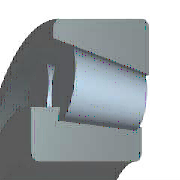
# Autodesk Inventor part: Подшипник 7205A ГОСТ 27365-87
Saved by Autodesk Inventor 2021 (Build 250183000, 183)
## iProperties
Created: 2020-01-21
Part Number: Подшипник 7205A ГОСТ 27365-87
Material: Сталь, мягкая
Description: Подшипники роликовые конические однорядные повышенной грузоподъемности
Document SubType Name: Modeling
Standard: ГОСТ 27365-87
Designer: gdevc
Standards Organization: GOST
Language: ru-RU
Size Designation: 7205A
Categories: <MemberInstance><Categories><Category DisplayName="Детали вала" InternalName="7f7aeb1f-a693-4053-b835-cee3144e0d98" Mnemonic="SHFT"><Category DisplayName="Подшипники" InternalName="242d30a3-7172-44e6-a363-b0a3d8f1b556" Mnemonic="BRNG"><CategoryParameter DisplayName="Ширина" InternalName="25fc5f6e-338b-4801-b5ed-8959743e396e" Mnemonic="wdth"/><CategoryParameter DisplayName="Обозначение размера" InternalName="2c4e891a-c8f4-49ed-a5c1-5131476c6feb" Mnemonic="sizedes"/><CategoryParameter DisplayName="Номинальная динамическая нагрузка" InternalName="440972dd-7009-4861-bd45-69ffbb461423" Mnemonic="bdynlrat"/><CategoryParameter DisplayName="Диаметр вала" InternalName="91302473-2833-4451-a660-c5d4a8d6a031" Mnemonic="shaftdia"/><CategoryParameter DisplayName="Угол касания" InternalName="aa21a452-7974-4a55-b5cf-1c2972de2aea" Mnemonic="TouchAngle"/><CategoryParameter DisplayName="Наружный диаметр" InternalName="d441686c-04bd-4681-b674-94fbc173ec23" Mnemonic="outdia"/><Category DisplayName="Подшипники роликовые" InternalName="a40a3fd7-d489-4921-9892-cb944902a182" Mnemonic="ROLLBEAR"><CategoryParameter DisplayName="Номинальная статическая нагрузка" InternalName="124ef669-bc53-497e-8b3b-9e9432584ac1" Mnemonic="bstatlrat"/><CategoryParameter DisplayName="Коэффициент радиальной динамической нагрузки при Fa/Fr &gt; e" InternalName="1feec4eb-3d91-4913-989d-fa96ab069f3d" Mnemonic="raddynfc2"/><CategoryParameter DisplayName="Коэффициент осевой динамической нагрузки при Fa/Fr &gt; e" InternalName="200b4357-faba-40fb-9da6-9412c8ddeb78" Mnemonic="axdynfc2"/><CategoryParameter DisplayName="Радиус" InternalName="2322b21e-a448-4b16-bf77-0b09a9a1e5fa" Mnemonic="rad"/><CategoryParameter DisplayName="Мин. диаметр вала" InternalName="27c639de-1f82-42cb-a17a-a84ebe509f1b" Mnemonic="minshaftdia"/><CategoryParameter DisplayName="Ограничивающая скорость смазка" InternalName="34ed7782-22cd-44b7-90f2-16a4b10c8234" Mnemonic="lubgrsp"/><CategoryParameter DisplayName="Масса" InternalName="35563771-cdde-4f36-b8ea-a6490dc90073" Mnemonic="mass"/><CategoryParameter DisplayName="Ограничивающее скорость масло" InternalName="576744bc-a99a-4f12-bf8b-8b83672ef882" Mnemonic="oilspd"/><CategoryParameter DisplayName="Коэффициент радиальной статической нагрузки" InternalName="646321f5-f93b-4aec-b962-0341aa1dcfaf" Mnemonic="raddynfc0"/><CategoryParameter DisplayName="Макс. радиус отсека скругления" InternalName="890763e8-95b6-457a-9b07-8de657924e40" Mnemonic="maxstprad"/><CategoryParameter DisplayName="Коэффициент осевой динамической нагрузки при Fa/Fr &lt;= e" InternalName="b1d498d2-5149-4618-b12c-23a3d5a7c887" Mnemonic="axdynfc1"/><CategoryParameter DisplayName="Коэффициент радиальной динамической нагрузки при Fa/Fr  &lt;= e" InternalName="b75e8b40-fb1d-483d-887b-ce2ffe1b5422" Mnemonic="raddynfc1"/><CategoryParameter DisplayName="Коэффициент трения" InternalName="ceddb76f-d381-429d-bef5-367584929fdf" Mnemonic="fricfct"/><CategoryParameter DisplayName="Коэффициент осевой статической нагрузки" InternalName="ea413b62-e115-405b-882c-23d570c3be21" Mnemonic="axdynfc0"/><CategoryParameter DisplayName="Граничное значение для определения коэффициента" InternalName="f0539972-a230-481a-8ae0-28002199c8fb" Mnemonic="limvalfac"/><CategoryParameter DisplayName="Ресурс" InternalName="f80a4cc4-8fb3-4eaa-808e-6f490e608712" Mnemonic="lifeexp"/><CategoryParameter DisplayName="Макс. диаметр отсека втулки" InternalName="feeea31f-2614-4692-af6e-a054e6e558b2" Mnemonic="maxhubdia"/><Category DisplayName="Подшипники роликовые конические" InternalName="326936b4-87e6-427a-a604-f9fe807308df" Mnemonic="RBTRB"/></Category></Category></Category><Category DisplayName="ТипДанных" InternalName="23b78d0f-2648-40c6-8793-ca6db495c9e8" Mnemonic="DATATYPE"><CategoryParameter DisplayName="ОтображаемоеИмя" InternalName="05415f3d-3907-474b-a020-eb9d644f4cf3" Mnemonic="DISPLAYNAME"/><CategoryParameter DisplayName="Стандарт" InternalName="0c0a119c-1e12-4c84-803f-101930972f5e" Mnemonic="STANDARD"/><CategoryParameter DisplayName="Наименование" InternalName="13903e3d-64b1-4950-80da-f627842ea37f" Mnemonic="DESCRIPTION"/><CategoryParameter DisplayName="Обозначение" InternalName="2675968c-4ce5-49e0-a4f5-552d29089031" Mnemonic="DESIGNATION"/><CategoryParameter DisplayName="Строка по умолчанию" InternalName="2af9ec52-faaa-4026-b378-f9fa4afca842" Mnemonic="DEFAULTROW"/><CategoryParameter DisplayName="Имя папки" InternalName="3f06958e-8713-4116-9be7-ed6184ecc97b" Mnemonic="FOLDERNAME"/><CategoryParameter DisplayName="Указатель редакций" InternalName="45a75005-10b1-4dfc-8d6d-dfe629f0b93c" Mnemonic="REVISIONGUID"/><CategoryParameter DisplayName="ИмяФайла" InternalName="8b46a4cc-9585-4fed-90c3-899f57e09a73" Mnemonic="FILENAME"/><CategoryParameter DisplayName="ОргСтанд" InternalName="8f5914e1-4693-403f-8ab5-d37768198c9d" Mnemonic="STDSORG"/><CategoryParameter DisplayName="Версия семейства" InternalName="914462f6-6e19-4b14-ba84-155b9680b1d0" Mnemonic="FAMILYREVISION"/><CategoryParameter DisplayName="Редакция стандарта" InternalName="91d5a463-65c2-4fde-b823-3b7fea5e8e17" Mnemonic="STANDARDREVISION"/><CategoryParameter DisplayName="редакция элемента" InternalName="a65d44b9-392f-4f4f-857b-e4b3d54996fe" Mnemonic="MEMBERREVISION"/><CategoryParameter DisplayName="ФорматКлипа" InternalName="bc51e27b-3422-4e78-93ef-cec197ddf230" Mnemonic="CLIPFORMAT"/><CategoryParameter DisplayName="Изготовитель" InternalName="cd6c7a72-a28a-4e50-99a9-2c7f4e13e5ad" Mnemonic="MANUFACTURER"/><CategoryParameter DisplayName="ВнутреннееИмя" InternalName="cf1d0246-76d9-4b4a-8305-fa0409afb5c1" Mnemonic="INTERNALNAME"/><CategoryParameter DisplayName="Метрическая" InternalName="e2385c5b-1ea4-4823-96a8-8de651266ec3" Mnemonic="ISMETRIC"/><Category DisplayName="Деталь" InternalName="c0e0b642-3bcb-4cc8-9e80-f96d35c4afa4" Mnemonic="PART"><CategoryParameter DisplayName="Номер детали" InternalName="016b6077-bfbe-49bd-92c9-d8d59c39c941" Mnemonic="PARTNUMBER"/><CategoryParameter DisplayName="Инвентарный номер" InternalName="4dba7c1c-e26c-444e-836c-b08b433409a8" Mnemonic="STOCKNUMBER"/><CategoryParameter DisplayName="Ключ материала" InternalName="5c9a8adb-dd2b-4535-b97f-0a94a95fe41f" Mnemonic="MATERIALKEY"/><CategoryParameter DisplayName="Материал" InternalName="818a152a-d3c3-49ca-80ee-df7d91421b8e" Mnemonic="MATERIAL"/></Category></Category></Categories><FamilyTemplate Id="Bearing GOST 27365-87"><FamilyTemplateParameters><FamilyTemplateParameter ObjectType="kUserParameterObject" ValueType="xs:double" Id="1" ObjectReferenceKey="Angle"/><FamilyTemplateParameter ObjectType="kUserParameterObject" ValueType="xs:double" Id="2" ObjectReferenceKey="B"/><FamilyTemplateParameter ObjectType="kUserParameterObject" ValueType="xs:double" Id="3" ObjectReferenceKey="C0_"/><FamilyTemplateParameter ObjectType="kUserParameterObject" ValueType="xs:double" Id="4" ObjectReferenceKey="C_"/><FamilyTemplateParameter ObjectType="kUserParameterObject" ValueType="xs:double" Id="5" ObjectReferenceKey="C__"/><FamilyTemplateParameter ObjectType="kUserParameterObject" ValueType="xs:double" Id="6" ObjectReferenceKey="d"/><FamilyTemplateParameter ObjectType="kUserParameterObject" ValueType="xs:double" Id="7" ObjectReferenceKey="D_"/><FamilyTemplateParameter ObjectType="kUserParameterObject" ValueType="xs:double" Id="8" ObjectReferenceKey="E_"/><FamilyTemplateParameter ObjectType="kUserParameterObject" ValueType="xs:double" Id="10" ObjectReferenceKey="r1_smin"/><FamilyTemplateParameter ObjectType="kUserParameterObject" ValueType="xs:double" Id="11" ObjectReferenceKey="r2_smin"/><FamilyTemplateParameter ObjectType="kUserParameterObject" ValueType="xs:double" Id="13" ObjectReferenceKey="T_"/><FamilyTemplateParameter ObjectType="kPropertyObject" ValueType="xs:string" Id="100" ObjectReferenceKey="{32853F0F-3444-11d1-9E93-0060B03C1CA6}" SubObjectId="52"/><FamilyTemplateParameter ObjectType="kPropertyObject" ValueType="xs:string" Id="105" ObjectReferenceKey="{32853F0F-3444-11d1-9E93-0060B03C1CA6}" SubObjectId="5"/><FamilyTemplateParameter ObjectType="kPartComponentDefinitionObject" ValueType="xs:string" Id="110" SubObjectId="Material"/><FamilyTemplateParameter ObjectType="kPropertyObject" ValueType="xs:string" Id="112" ObjectReferenceKey="{F29F85E0-4FF9-1068-AB91-08002B27B3D9}" SubObjectId="2"/></FamilyTemplateParameters></FamilyTemplate><CategoryParameterMap><ParamToTemplateMap><ParamToTemplate CategoryParameter="//CategoryParameter[@InternalName='05415f3d-3907-474b-a020-eb9d644f4cf3']" ConstantValue="Bearing GOST 27365-87"/><ParamToTemplate CategoryParameter="//CategoryParameter[@InternalName='0c0a119c-1e12-4c84-803f-101930972f5e']" ConstantValue="GOST 27365-87"/><ParamToTemplate CategoryParameter="//CategoryParameter[@InternalName='13903e3d-64b1-4950-80da-f627842ea37f']" ConstantValue="Single-row tapered roller bearings of extra load ratings"/><ParamToTemplate CategoryParameter="//CategoryParameter[@InternalName='2af9ec52-faaa-4026-b378-f9fa4afca842']" ConstantValue="1"/><ParamToTemplate CategoryParameter="//CategoryParameter[@InternalName='3f06958e-8713-4116-9be7-ed6184ecc97b']" ConstantValue="Bearing GOST 27365-87"/><ParamToTemplate CategoryParameter="//CategoryParameter[@InternalName='45a75005-10b1-4dfc-8d6d-dfe629f0b93c']" ConstantValue="7538fd77-6ae2-4b7c-85b1-12ee0fb3b084"/><ParamToTemplate CategoryParameter="//CategoryParameter[@InternalName='8f5914e1-4693-403f-8ab5-d37768198c9d']" ConstantValue="GOST"/><ParamToTemplate CategoryParameter="//CategoryParameter[@InternalName='914462f6-6e19-4b14-ba84-155b9680b1d0']" ConstantValue="11"/><ParamToTemplate CategoryParameter="//CategoryParameter[@InternalName='91d5a463-65c2-4fde-b823-3b7fea5e8e17']" TemplateParameter="103"/><ParamToTemplate CategoryParameter="//CategoryParameter[@InternalName='bc51e27b-3422-4e78-93ef-cec197ddf230']" ConstantValue="CF_INVENTOR.STDPARTS"/><ParamToTemplate CategoryParameter="//CategoryParameter[@InternalName='cd6c7a72-a28a-4e50-99a9-2c7f4e13e5ad']" TemplateParameter="104"/><ParamToTemplate CategoryParameter="//CategoryParameter[@InternalName='cf1d0246-76d9-4b4a-8305-fa0409afb5c1']" ConstantValue="7d777af1-58f4-4436-bd59-163e675d2302"/><ParamToTemplate CategoryParameter="//CategoryParameter[@InternalName='e2385c5b-1ea4-4823-96a8-8de651266ec3']" ConstantValue="true"/><ParamToTemplate CategoryParameter="//CategoryParameter[@InternalName='8b46a4cc-9585-4fed-90c3-899f57e09a73']" ConstantValue="Подшипник 7205A ГОСТ 27365-87"/><ParamToTemplate CategoryParameter="//CategoryParameter[@InternalName='a65d44b9-392f-4f4f-857b-e4b3d54996fe']" ConstantValue="0a9fa57e-6a9e-4d45-9e98-71951d08c575"/><ParamToTemplate CategoryParameter="//CategoryParameter[@InternalName='2675968c-4ce5-49e0-a4f5-552d29089031']" TemplateParameter="100"/><ParamToTemplate CategoryParameter="//CategoryParameter[@InternalName='2c4e891a-c8f4-49ed-a5c1-5131476c6feb']" TemplateParameter="100"/><ParamToTemplate CategoryParameter="//CategoryParameter[@InternalName='d441686c-04bd-4681-b674-94fbc173ec23']" TemplateParameter="7"/><ParamToTemplate CategoryParameter="//CategoryParameter[@InternalName='818a152a-d3c3-49ca-80ee-df7d91421b8e']" TemplateParameter="110"/><ParamToTemplate CategoryParameter="//CategoryParameter[@InternalName='016b6077-bfbe-49bd-92c9-d8d59c39c941']" TemplateParameter="105"/><ParamToTemplate CategoryParameter="//CategoryParameter[@InternalName='25fc5f6e-338b-4801-b5ed-8959743e396e']" TemplateParameter="13"/><ParamToTemplate CategoryParameter="//CategoryParameter[@InternalName='91302473-2833-4451-a660-c5d4a8d6a031']" TemplateParameter="6"/></ParamToTemplateMap></CategoryParameterMap></MemberInstance>
Density: 7.85 g/cm^3
Appearance: С умеренной полировкой
IsCustomPart: 1
Title: Подшипник
Author: gdevc
Autodesk Inventor part; units mm, degrees
ref_plane "YZ Plane" through (0, 0, 0) normal (1, 0, 0) x (0, 1, 0)
ref_plane "XZ Plane" through (0, 0, 0) normal (0, 1, 0) x (-1, 0, 0)
ref_plane "XY Plane" through (0, 0, 0) normal (0, 0, 1) x (1, 0, 0)
sketch "Sketch1" plane through (0, 0, 0) normal (0, 0, 1) x (1, 0, 0)
  line L0 (-2.486985, 0) -> (14.486985, 0) construction
  line L1 (0, -3.712426) -> (0, 22.274559) construction
  line L2 (1, 26) -> (12, 26)
  arc A0 (13, 25) -> (12, 26) centre (12, 25) ccw
  line L3 (13, 25) -> (13, 23.817441)
  line L4 (13, 23.817441) -> (0, 20.5675)
  line L5 (0, 20.5675) -> (0, 25)
  line L6 (2.25, 12.5) -> (15.25, 12.5)
  line L7 (16.25, 13.5) -> (16.25, 16.9)
  line L8 (12.906383, 16.82) -> (1.25, 15.5)
  line L9 (1.777201, 18.253118) -> (12.303191, 20.156224)
  line L10 (1.3, 20.892494) -> (2.254402, 15.613741)
  line L11 (11.7, 23.492447) -> (12.906383, 16.82)
  arc A1 (1, 26) -> (0, 25) centre (1, 25) ccw
  line L12 (0, 20.5675) -> (3.750515, 20.5675) construction
  arc A2 (15.25, 12.5) -> (16.25, 13.5) centre (15.25, 13.5) ccw
  line L13 (1.25, 15.5) -> (1.25, 13.5)
  arc A3 (1.25, 13.5) -> (2.25, 12.5) centre (2.25, 13.5) ccw
  line L14 (12.711118, 17.9) -> (15.25, 17.9)
  arc A4 (16.25, 16.9) -> (15.25, 17.9) centre (15.25, 16.9) ccw
  point P0 (0, 0)
  dimension "d0" = 1
  dimension "d1" = 1
  dimension "d2" = 13
  dimension "d5" = 16.25
  dimension "d6" = 15
  dimension "d7" = 52
  dimension "d8" = 25
  dimension "d9" = 41.135
  dimension "d10" = 14.036
  dimension "d11" = 5.4
  dimension "d12" = 3
  dimension "d13" = 1.3
  dimension "d14" = 1.3
  dimension "d15" = 1.08
  constraints: 26 end point, 11 point on circle, 10 tangent, 5 centre point, 5 perpendicular, 5 point on line, 4 midpoint, 3 equal radius, 2 parallel, 2 vertical, 1 collinear, 1 other
  measures "d0" radius of A1
  measures "d1" radius of A2
  measures "d2" distance between parallel lines of L3 L5
  measures "d5" distance between parallel lines of L5 L7
  measures "d6" distance between parallel lines of L7 L13
  measures "d7" diameter of L2 L0
  measures "d8" diameter of L6 L0
  measures "d9" diameter of L4.end L0
  measures "d10" angle of L4 L12
  measures "d11" distance between parallel lines of L6 L14
  measures "d12" distance from line of L6 L8.end
  measures "d13" distance from line of L3 L11.start
  measures "d14" distance from line of L5 L10.start
  measures "d15" distance from line of L14 L8.start
revolve "Вращение1" add sketch "Sketch1" angle 360 about axis through (-10, 0, 0) along (1, 0, 0) contours L2 A0 L3 L4 L5 A1 | L8 L11 L14 A4 L7 A2 L6 A3 L13
revolve "Вращение2" add sketch "Sketch1" angle 360 about axis through (1.777201, 18.253118, 0) along (0.9840457, 0.1779161, 0) contours L4 L11 L9 L10
pattern_circular "Круговой Массив1" count 9 over 360 about axis through (-10, 0, 0) along (1, 0, 0) of "Вращение2"
equation "\"d0\" = r2_smin"
equation "\"d1\" = r1_smin"
equation "\"d2\" = C_"
equation "\"d5\" = T_"
equation "\"d6\" = B"
equation "\"d7\" = D_"
equation "\"d8\" = d"
equation "\"d9\" = E_"
equation "\"d10\" = Angle"
equation "\"d11\" = -0.2 * d + 0.2 * D_"
equation "\"d12\" = -0.111111 * d + 0.111111 * D_"
equation "\"d13\" = 0.1 * d2"
equation "\"d14\" = d13"
equation "\"d15\" = 0.2 * d11"
equation "\"d\" = 25"
equation "\"D_\" = 52"
equation "\"B\" = 15"
equation "\"C_\" = 13"
equation "\"T_\" = 16.25"
equation "\"Angle\" = 14.036deg"
equation "\"E_\" = 41.135"
equation "\"r1_smin\" = 1"
equation "\"r2_smin\" = 1"
body "Solid1"
